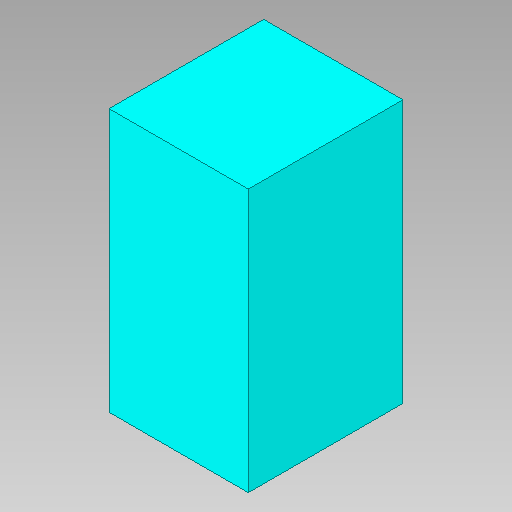
# Autodesk Inventor part: CHIP-LED0603
Saved by Autodesk Inventor 2020.1 (Build 241239000, 239)
## iProperties
Created: 2015-11-24
Part Number: CHIP-LED0603
Material: Generic
Document SubType Name: Modeling
Designer: PhillipD
Density: 1 g/cm^3
Appearance: CHIP-LED0603, CHIP-LED0603
Author: PhillipD
Autodesk Inventor part; units mm, degrees
ref_plane "YZ Plane" through (0, 0, 0) normal (1, 0, 0) x (0, 1, 0)
ref_plane "XZ Plane" through (0, 0, 0) normal (0, 1, 0) x (-1, 0, 0)
ref_plane "XY Plane" through (0, 0, 0) normal (0, 0, 1) x (1, 0, 0)
sketch "CHIP-LED0603, CHIP-LED0603_86" plane through (0, 0, 0) normal (0, 0, 1) x (1, 0, 0)
  line L0 (-0.4508, 0.85) -> (0.45, 0.85)
  line L1 (0.45, 0.85) -> (0.45, -0.85)
  line L2 (0.45, -0.85) -> (-0.4508, -0.85)
  line L3 (-0.4508, -0.85) -> (-0.4508, 0.85)
  constraints: 8 end point
extrude "Extrusion1" add sketch "CHIP-LED0603, CHIP-LED0603_86" along normal blind 1
body "Solid1"
